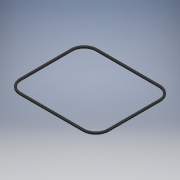
# Autodesk Inventor part: PayloadGermination_Seal
Saved by Autodesk Inventor 2018 (Build 220112000, 112)
## iProperties
Created: 2018-07-29
Part Number: PayloadGermination_Seal
Material: Rubber
Document SubType Name: Modeling
Designer: Bradley
Density: 0.93 g/cm^3
Appearance: Rubber - Black
Author: Bradley
Autodesk Inventor part; units mm, degrees
ref_plane "YZ Plane" through (0, 0, 0) normal (1, 0, 0) x (0, 1, 0)
ref_plane "XZ Plane" through (0, 0, 0) normal (0, 1, 0) x (-1, 0, 0)
ref_plane "XY Plane" through (0, 0, 0) normal (0, 0, 1) x (1, 0, 0)
sketch "Sketch1" plane through (0, 0, 0) normal (0, 0, 1) x (1, 0, 0)
  line L0 (-29.5, -34.6) -> (29.5, -34.6)
  line L1 (40.1, -24) -> (40.1, 24)
  line L2 (29.5, 34.6) -> (-29.5, 34.6)
  line L3 (-40.1, 24) -> (-40.1, -24)
  line L4 (-40.1, -34.6) -> (40.1, 34.6) construction
  line L5 (40.1, -34.6) -> (-40.1, 34.6) construction
  arc A0 (-29.5, 34.6) -> (-40.1, 24) centre (-29.5, 24) ccw
  arc A1 (-40.1, -24) -> (-29.5, -34.6) centre (-29.5, -24) ccw
  arc A2 (29.5, -34.6) -> (40.1, -24) centre (29.5, -24) ccw
  arc A3 (40.1, 24) -> (29.5, 34.6) centre (29.5, 24) ccw
  point P0 (0, 0)
  dimension "d0" = 69.2
  dimension "d1" = 80.2
  dimension "d2" = 10.6
  constraints: 12 end point, 8 point on circle, 8 point on line, 8 tangent, 4 centre point, 3 equal radius, 2 midpoint, 2 parallel, 1 horizontal, 1 perpendicular
  measures "d0" distance of L5.end L4.start
  measures "d1" distance of L4.end L5.end
  measures "d2" radius of A0
sketch "Sketch2" plane through (0, 0, 0) normal (0, 1, 0) x (-1, 0, 0)
  line L0 (41.7614, 0.75) -> (40.4386, 0.75)
  arc A0 (40.4386, 0.75) -> (40.4386, -0.75) centre (41.1, 0) ccw
  arc A1 (41.7614, -0.75) -> (41.7614, 0.75) centre (41.1, 0) ccw
  line L1 (41.7614, -0.75) -> (40.4386, -0.75)
  point P0 (0, 0)
  point P1 (40.1, 0)
  point P2 (40.1, 0)
  point P3 (40.1, 0)
  point P4 (41.1, 0.75)
  dimension "d3" = 1.5
  dimension "d4" = 1
  constraints: 5 point on circle, 4 end point, 2 centre point, 2 horizontal, 1 concentric, 1 horizontal alignment, 1 midpoint, 1 parallel, 1 vertical alignment
  measures "d3" distance between parallel lines of L1 L0
  measures "d4" radius of A1
sweep "Sweep1" add profiles "Sketch2" path "Sketch1"
body "Solid1"
